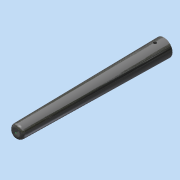
# Autodesk Inventor part: AntennaMast
Saved by Autodesk Inventor 2011 SP1 (Build 150282100, 282)
## iProperties
Created: 2011-08-14
Part Number: AntennaMast
Document SubType Name: Modeling
Designer: dgitz
Density: 1 g/cm^3
Author: dgitz
Autodesk Inventor part; units mm, degrees
sketch "Sketch1" plane through (0, 0, 0) normal (0, 0, 1) x (1, 0, 0)
  point P0 (0, 0)
sketch "Sketch2" plane through (0, 0, 0) normal (0, 0, 1) x (1, 0, 0)
  circle A0 centre (0, 0) radius 3.683
  dimension "d0" = 7.366
  constraints: 1 centre point, 1 coincident
  measures "d0" diameter of A0
ref_plane "Work Plane1" through (0, 0, -83.82) normal (0, 0, 1) x (1, 0, 0)
sketch "Sketch3" plane through (0, 0, -83.82) normal (0, 0, 1) x (1, 0, 0)
  circle A0 centre (0, 0) radius 4.826
  dimension "d2" = 9.652
  constraints: 1 centre point, 1 coincident
  measures "d2" diameter of A0
loft "Loft1" add profiles "Sketch2", "Sketch3"
fillet "Fillet1" radius 1.5875 1 edges at (-3.683, 0, 0)
ref_plane "Work Plane2" through (0, 4.826, 0) normal (0, 1, 0) x (-1, 0, 0)
sketch "Sketch4" plane through (0, 4.826, 0) normal (0, 1, 0) x (-1, 0, 0)
  circle A0 centre (0, -78.74) radius 0.8255
  line L0 (4.826, -83.82) -> (-4.826, -83.82) projected
  point P0 (0, 0)
  dimension "d9" = 1.651
  dimension "d10" = 5.08
  constraints: 1 centre point
  measures "d9" diameter of A0
  measures "d10" distance from line of L0 A0.centre
extrude "Extrusion1" cut sketch "Sketch4" against normal up to next
ref_plane "Work Plane3" through (4.826, 0, 0) normal (1, 0, 0) x (0, 1, 0)
body "Solid1"
